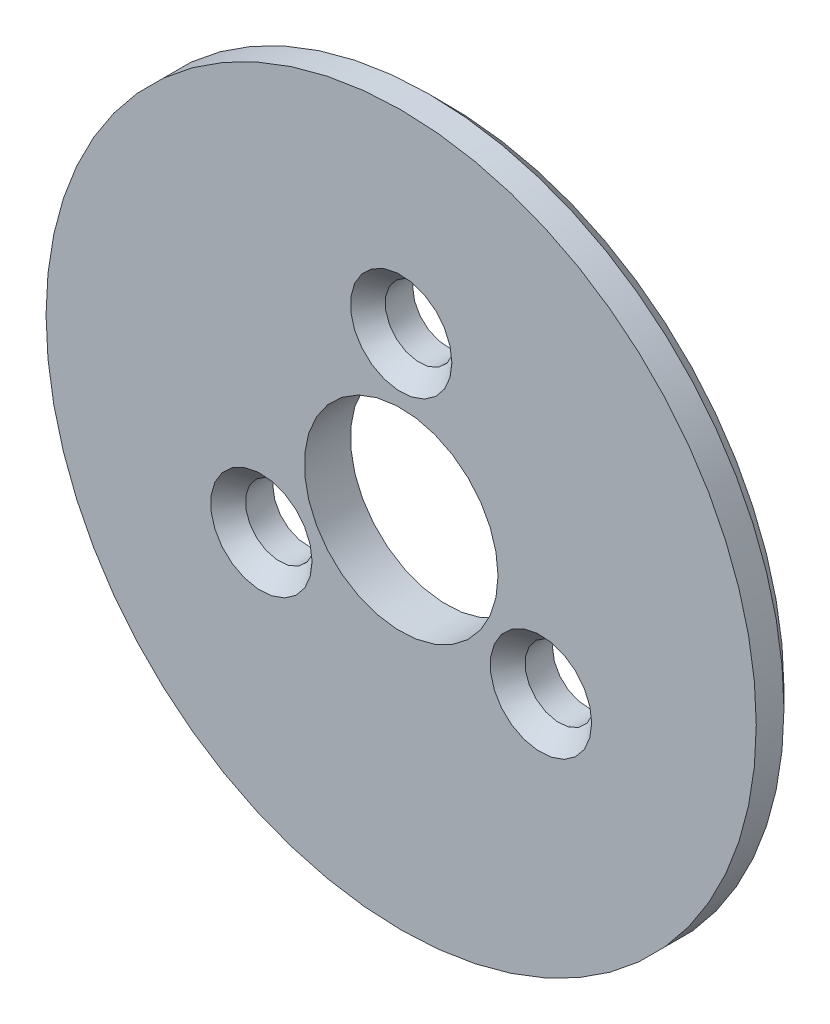
# Autodesk Inventor part: INNER_TIMING_PULLEY_COVER
Saved by Autodesk Inventor 2019.4 (Build 234330000, 330)
## iProperties
Created: 2019-11-13
Part Number: INNER_TIMING_PULLEY_COVER
Material: 一般
Document SubType Name: Modeling
Designer: y6tada
Density: 1 g/cm^3
Appearance: 既定
Author: y6tada
Autodesk Inventor part; units mm, degrees
ref_plane "YZ Plane" through (0, 0, 0) normal (1, 0, 0) x (0, 1, 0)
ref_plane "XZ Plane" through (0, 0, 0) normal (0, 1, 0) x (-1, 0, 0)
ref_plane "XY Plane" through (0, 0, 0) normal (0, 0, 1) x (1, 0, 0)
sketch "スケッチ1" plane through (0, 0, 0) normal (0, 0, 1) x (1, 0, 0)
  circle A0 centre (0, 0) radius 7.7
  circle A1 centre (0, 0) radius 2.1
  dimension "d0" = 4.2
  dimension "d1" = 15.4
  constraints: 2 centre point, 2 coincident
  measures "d0" diameter of A1
  measures "d1" diameter of A0
extrude "押し出し1" add sketch "スケッチ1" along normal blind 1
chamfer "面取り1" distance 0.4 angle 45 1 edges at (-7.7, 0, 0)
sketch "スケッチ2" plane through (0, 0, 1) normal (0, 0, 1) x (1, 0, 0)
  circle A0 centre (0, 3.5) radius 0.5915 construction
  point P0 (0, 0)
  point P1 (-3.0311, -1.75)
  point P2 (3.0311, -1.75)
  dimension "d9" = 360
  constraints: 1 coincident, 4 other
hole "穴1" at (0, 3.5, 1) at (-3.0311, -1.75, 1) at (3.0311, -1.75, 1) direction (0, 0, -1) diameter 1.5 end through all countersink diameter 2.2 countersink angle 82
